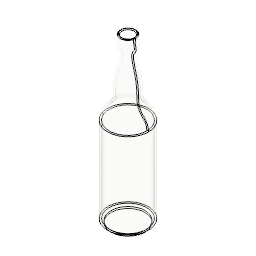
Soda_Bottle (Autodesk Fusion 360 design; units mm, degrees)
part number: 2026-02-11-10-47-13-960
Autodesk Fusion 360 part; units mm, degrees
sketch "Sketch1" plane through (0, 0, 0) normal (0, 0, 1) x (1, 0, 0)
  line L0 (0, 0) -> (0, 240)
  line L1 (0, 0) -> (30, 0)
  line L2 (30, 0) -> (30, 130)
  spline S0 degree 5 poles (30, 130) (30, 130.4916) (29.9839, 131.468) (29.9116, 132.9118) (29.704, 134.7945) (29.1841, 137.0746) (28.325, 139.2825) (27.0781, 141.426) (25.4631, 143.5242) (23.5923, 145.6106) (21.6303, 147.7292) (19.7624, 149.9322) (18.1589, 152.2777) (16.9439, 154.8263) (16.1539, 157.639) (15.7358, 160.7731) (15.5783, 164.2754) (15.5346, 168.1764) (15.4476, 172.4844) (15.1742, 177.179) (14.6107, 182.205) (13.7155, 187.4664) (12.5401, 192.817) (11.2138, 198.0754) (9.9084, 203.0492) (8.8109, 207.5569) (8.0917, 211.4506) (7.876, 214.6379) (8.2115, 217.1066) (9.043, 218.9429) (10.1687, 220.3666) (11.2535, 221.7141) (11.9722, 223.3043) (12.1093, 225.343) (11.7134, 227.7764) (11.0575, 230.332) (10.4811, 232.6734) (10.2706, 234.5183) (10.5195, 235.776) (11.0083, 236.6661) (11.3947, 237.5293) (11.4362, 238.3832) (11.2883, 239.1442) (11.1094, 239.7057) (11, 240) knots 0 0 0 0 0 0 0.025 0.05 0.075 0.1 0.125 0.15 0.175 0.2 0.225 0.25 0.275 0.3 0.325 0.35 0.375 0.4 0.425 0.45 0.475 0.5 0.525 0.55 0.575 0.6 0.625 0.65 0.675 0.7 0.725 0.75 0.775 0.8 0.825 0.85 0.875 0.9 0.925 0.95 0.975 1 1 1 1 1 1
  line L3 (30, 117.9219) -> (30, 142.0781)
  line L4 (0, 240) -> (11, 240)
  point P0 (27.2431, 141.0233)
  point P1 (17.6456, 153.4898)
  point P2 (14.3037, 183.7627)
  point P3 (8.8142, 218.2679)
  point P4 (11.9511, 224.1495)
  point P5 (10.3826, 234.3442)
  point P6 (11.1668, 237.0889)
  dimension "d1" = 240
  dimension "d2" = 30
  dimension "d3" = 130
  dimension "d7" = 11
  constraint coincident L0.start L1.start
  constraint vertical L0
  constraint perpendicular L0 L1
  constraint perpendicular L1 L2
  constraint midpoint L2.end L3
  constraint vertical L3
  constraint perpendicular L0 L4
  measures "d1" distance of L0.start L0.end
  measures "d2" distance of L0.start L1.end
  measures "d3" distance of L1.end L2.end
  measures "d7" distance of L0.end S0.end
revolve "Revolve1" add sketch "Sketch1" angle 360 about axis through (0, 0, 0) along (0, 1, 0)
fillet "Fillet1" radius 5 1 edges at (-27.9698, 0, -10.8485)
shell "Shell1" thickness 2.5 removed faces 1 at (-3.2467, 240, 0.051)
fillet "Fillet2" radius 1 2 edges at (-8.3327, 240, 0.0036) (-10.2556, 240, -3.9778)
